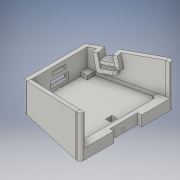
# Autodesk Inventor part: PIUBaseCaseV2
Saved by Autodesk Inventor 2016 (Build 200138000, 138)
## iProperties
Created: 2015-11-04
Part Number: PIUBaseCaseV2
Material: ABS Plastic
Document SubType Name: Modeling
Designer: jonathan
Density: 1.06 g/cm^3
Appearance: Smooth - White
Author: jonathan
Autodesk Inventor part; units mm, degrees
ref_plane "YZ Plane" through (0, 0, 0) normal (1, 0, 0) x (0, 1, 0)
ref_plane "XZ Plane" through (0, 0, 0) normal (0, 1, 0) x (-1, 0, 0)
ref_plane "XY Plane" through (0, 0, 0) normal (0, 0, 1) x (1, 0, 0)
sketch "Sketch1" plane through (0, 0, 0) normal (0, 1, 0) x (-1, 0, 0)
  line L0 (0, 27.305) -> (0, -27.305)
  line L1 (0, 0) -> (-62.23, 0)
  line L2 (-62.23, 41.6814) -> (-62.23, -41.6814)
  line L3 (0, 27.305) -> (-62.23, 41.6814)
  line L4 (0, -27.305) -> (-62.23, -41.6814)
  line L5 (0, -27.305) -> (3.81, -27.305)
  line L6 (3.81, -27.305) -> (3.81, -31.115)
  line L7 (3.81, -31.115) -> (0, -31.115)
  line L8 (0, -31.115) -> (0, -27.305)
  line L9 (0, 27.305) -> (3.81, 27.305)
  line L10 (3.81, 27.305) -> (3.81, 31.115)
  line L11 (3.81, 31.115) -> (0, 31.115)
  line L12 (0, 31.115) -> (0, 27.305)
  line L13 (-62.23, -41.6814) -> (-66.04, -41.6814)
  line L14 (-66.04, -41.6814) -> (-66.04, -45.4914)
  line L15 (-66.04, -45.4914) -> (-62.23, -45.4914)
  line L16 (-62.23, -45.4914) -> (-62.23, -41.6814)
  line L17 (-62.23, 41.6814) -> (-66.04, 41.6814)
  line L18 (-66.04, 41.6814) -> (-66.04, 45.4914)
  line L19 (-66.04, 45.4914) -> (-62.23, 45.4914)
  line L20 (-62.23, 45.4914) -> (-62.23, 41.6814)
  line L21 (3.81, 27.305) -> (3.81, -27.305)
  line L22 (0, -31.115) -> (-62.23, -45.4914)
  line L23 (-66.04, -41.6814) -> (-66.04, 41.6814)
  line L24 (-62.23, 45.4914) -> (0, 31.115)
  dimension "d0" = 54.61
  dimension "d1" = 62.23
  dimension "d2" = 83.3628
  dimension "d3" = 3.81
  dimension "d4" = 3.81
  dimension "d5" = 3.81
  dimension "d6" = 3.81
  dimension "d7" = 3.81
  dimension "d8" = 3.81
  dimension "d9" = 3.81
  dimension "d10" = 3.81
  constraints: 50 end point, 8 parallel, 5 horizontal, 4 perpendicular, 2 midpoint, 2 vertical, 1 coincident
  measures "d0" distance of L0.start L0.end
  measures "d1" distance of L1.end L1.start
  measures "d2" distance of L2.start L2.end
  measures "d3" distance of L6.end L7.end
  measures "d4" distance of L5.end L6.end
  measures "d5" distance of L11.end L10.end
  measures "d6" distance of L10.end L9.end
  measures "d7" distance of L15.end L14.end
  measures "d8" distance of L14.end L13.end
  measures "d9" distance of L18.end L19.end
  measures "d10" distance of L17.end L18.end
extrude "Extrusion1" add sketch "Sketch1" along normal blind 3.81 contours L0 L1 L2 L3 | L0 L4 L2 L1
sketch "Sketch2" plane through (0, 0, 0) normal (0, -1, 0) x (1, 0, 0)
  line L0 (0, -27.305) -> (0, 27.305) projected
  line L1 (0, 27.305) -> (-3.81, 27.305)
  line L2 (-3.81, 27.305) -> (-3.81, 31.115)
  line L3 (-3.81, 31.115) -> (0, 31.115)
  line L4 (0, 31.115) -> (0, 27.305)
  line L5 (0, -27.305) -> (-3.81, -27.305)
  line L6 (-3.81, -27.305) -> (-3.81, -31.115)
  line L7 (-3.81, -31.115) -> (0, -31.115)
  line L8 (0, -31.115) -> (0, -27.305)
  line L9 (62.23, 41.6814) -> (62.23, -41.6814) projected
  line L10 (62.23, -41.6814) -> (66.04, -41.6814)
  line L11 (66.04, -41.6814) -> (66.04, -45.4914)
  line L12 (66.04, -45.4914) -> (62.23, -45.4914)
  line L13 (62.23, -45.4914) -> (62.23, -41.6814)
  line L14 (62.23, 41.6814) -> (66.04, 41.6814)
  line L15 (66.04, 41.6814) -> (66.04, 45.4914)
  line L16 (66.04, 45.4914) -> (62.23, 45.4914)
  line L17 (62.23, 45.4914) -> (62.23, 41.6814)
  line L18 (-3.81, 27.305) -> (-3.81, -27.305)
  point P0 (0, 0)
  dimension "d13" = 3.81
  dimension "d14" = 3.81
  dimension "d15" = 3.81
  dimension "d16" = 3.81
  dimension "d17" = 3.81
  dimension "d18" = 3.81
  dimension "d19" = 3.81
  dimension "d20" = 3.81
  constraints: 34 end point, 8 parallel, 4 horizontal, 4 perpendicular
  measures "d13" distance of L2.end L3.end
  measures "d14" distance of L1.end L2.end
  measures "d15" distance of L7.end L6.end
  measures "d16" distance of L6.end L5.end
  measures "d17" distance of L11.end L12.end
  measures "d18" distance of L10.end L11.end
  measures "d19" distance of L16.end L15.end
  measures "d20" distance of L15.end L14.end
extrude "Extrusion2" add sketch "Sketch2" against normal blind 25.4 contours L5 L18 L1 L0 | L8 L7 L6 L5 | L1 L2 L3 L4
sketch "Sketch3" plane through (0, 0, 0) normal (0, -1, 0) x (1, 0, 0)
  line L0 (62.23, 41.6814) -> (62.23, -41.6814) projected
  line L1 (62.23, -41.6814) -> (66.04, -41.6814)
  line L2 (66.04, -41.6814) -> (66.04, -45.4914)
  line L3 (66.04, -45.4914) -> (62.23, -45.4914)
  line L4 (62.23, -45.4914) -> (62.23, -41.6814)
  line L5 (62.23, 41.6814) -> (66.04, 41.6814)
  line L6 (66.04, 41.6814) -> (66.04, 45.4914)
  line L7 (66.04, 45.4914) -> (62.23, 45.4914)
  line L8 (62.23, 45.4914) -> (62.23, 41.6814)
  line L9 (66.04, -41.6814) -> (66.04, 41.6814)
  point P0 (0, 0)
  dimension "d23" = 3.81
  dimension "d24" = 3.81
  dimension "d25" = 3.81
  dimension "d26" = 3.81
  constraints: 18 end point, 4 parallel, 2 horizontal, 2 perpendicular
  measures "d23" distance of L2.end L3.end
  measures "d24" distance of L1.end L2.end
  measures "d25" distance of L7.end L6.end
  measures "d26" distance of L6.end L5.end
extrude "Extrusion3" add sketch "Sketch3" against normal blind 38.1
sketch "Sketch4" plane through (0, 3.81, 0) normal (0, 1, 0) x (1, 0, 0)
  point P0 (0, 0)
sketch "Sketch5" plane through (0, 0, 27.305) normal (-0.2250919, 0, 0.9743375) x (0.9743375, 0, 0.2250919)
  line L0 (0, 3.81) -> (63.869, 3.81) projected
  line L1 (0, 0) -> (0, 3.81) projected
  line L2 (63.869, 3.81) -> (0, 3.81)
  line L3 (0, 3.81) -> (0, 0)
  line L4 (0, 0) -> (63.869, 0)
  line L5 (63.869, 0) -> (63.869, 3.81)
  line L6 (63.869, 3.81) -> (63.869, 38.1)
  line L7 (0, 3.81) -> (0, 25.4)
  line L8 (0, 25.4) -> (63.869, 38.1)
  point P0 (-6.1461, 0)
  dimension "d29" = 34.29
  dimension "d34" = 21.59
  constraints: 14 end point, 2 parallel, 2 vertical, 1 horizontal, 1 perpendicular
  measures "d29" distance of L0.end L6.end
  measures "d34" distance of L2.end L7.end
extrude "Extrusion4" add sketch "Sketch5" along normal blind 3.81
sketch "Sketch6" plane through (0, 0, 0) normal (0, -1, 0) x (1, 0, 0)
  line L0 (62.23, 41.6814) -> (62.23, -41.6814) projected
  line L1 (62.23, 45.4914) -> (62.23, 41.6814) projected
  line L2 (62.23, 41.6814) -> (62.23, 45.4914)
  line L3 (-0.4344, 31.115) -> (61.3724, 45.3936) projected
  line L4 (62.23, 45.4914) -> (61.3724, 45.3936)
  line L5 (61.3724, 45.3936) -> (62.23, 41.6814)
  point P0 (0, 0)
  constraints: 6 end point, 1 collinear, 1 perpendicular
extrude "Extrusion5" add sketch "Sketch6" against normal blind 38.1
sketch "Sketch7" plane through (0, 0, -27.305) normal (-0.2250919, 0, -0.9743375) x (-0.9743375, 0, 0.2250919)
  point P0 (6.1461, 0)
sketch "Sketch8" plane through (0, 0, -27.305) normal (-0.2250919, 0, -0.9743375) x (-0.9743375, 0, 0.2250919)
  line L0 (-63.869, 0) -> (-63.869, 3.81) projected
  line L1 (-63.869, 3.81) -> (-63.869, 38.1)
  line L2 (-63.869, 3.81) -> (0, 3.81) projected
  line L3 (0, 3.81) -> (0, 25.4)
  line L4 (0, 3.81) -> (-63.869, 3.81)
  line L5 (-63.869, 38.1) -> (0, 25.4)
  point P0 (6.1461, 0)
  dimension "d35" = 34.29
  dimension "d36" = 21.59
  constraints: 8 end point, 2 vertical, 1 collinear
  measures "d35" distance of L0.end L1.end
  measures "d36" distance of L2.end L3.end
extrude "Extrusion6" add sketch "Sketch8" along normal blind 3.81
sketch "Sketch9" plane through (0, 0, 0) normal (0, -1, 0) x (1, 0, 0)
  line L0 (62.23, -45.4914) -> (62.23, -41.6814) projected
  line L1 (-0.4344, -31.115) -> (-3.81, -31.115) projected
  line L2 (-3.81, -31.115) -> (0, -31.115) projected
  line L3 (-0.4344, -31.115) -> (0, -31.115)
  line L4 (0, 27.305) -> (0, -27.305) projected
  line L5 (0, -31.115) -> (0, -27.305)
  line L6 (0, -27.305) -> (62.23, -41.6814)
  line L7 (62.23, -41.6814) -> (61.3724, -45.3936) projected
  line L8 (62.23, -45.4914) -> (61.3724, -45.3936)
  line L9 (61.3724, -45.3936) -> (-0.4344, -31.115)
  line L10 (-0.8576, -31.0172) -> (61.3724, -45.3936) projected
  point P0 (0, 0)
  constraints: 10 end point, 1 collinear, 1 horizontal, 1 perpendicular
extrude "Extrusion7" add sketch "Sketch9" against normal blind 3.81 contours L7 L9 L2 L5 L6
sketch "Sketch10" plane through (0, 0, 0) normal (0, -1, 0) x (1, 0, 0)
  line L0 (0, -27.305) -> (62.23, -41.6814) projected
  line L1 (62.23, -41.6814) -> (62.23, -45.4914)
  line L2 (-0.4344, -31.115) -> (61.3724, -45.3936) projected
  line L3 (62.23, -45.4914) -> (61.3724, -45.3936)
  line L4 (62.23, -41.6814) -> (61.3724, -45.3936) projected
  line L5 (61.3724, -45.3936) -> (62.23, -41.6814)
  point P0 (0, 0)
  constraints: 6 end point, 1 collinear, 1 vertical
extrude "Extrusion8" add sketch "Sketch10" against normal blind 38.1
sketch "Sketch11" plane through (0, 3.81, 0) normal (0, 1, 0) x (1, 0, 0)
  line L0 (62.23, 41.6814) -> (0, 27.305) projected
  line L1 (62.23, -41.6814) -> (62.23, 41.6814) projected
  line L2 (62.23, 41.6814) -> (62.23, -41.6814)
  line L3 (0, -27.305) -> (62.23, -41.6814) projected
  line L4 (62.23, -41.6814) -> (0, -27.305)
  line L5 (0, 27.305) -> (0, -27.305)
  line L6 (62.23, 41.6814) -> (62.23, -41.6814) projected
  line L7 (62.23, 41.6814) -> (0, 27.305)
  line L8 (62.23, 41.6814) -> (58.277, 36.7118)
  line L9 (62.23, 41.6814) -> (68.58, 41.6814) construction
  line L10 (62.23, -41.6814) -> (58.277, -36.7118)
  line L11 (62.23, -41.6814) -> (68.58, -41.6814) construction
  line L12 (0, 27.305) -> (4.9703, 23.3529)
  line L13 (0, 27.305) -> (6.35, 27.305) construction
  line L14 (0, -27.305) -> (4.9703, -23.3529)
  line L15 (0, -27.305) -> (6.35, -27.305) construction
  line L16 (4.9703, -23.3529) -> (4.9703, 23.3529)
  line L17 (58.277, 36.7118) -> (4.9703, 23.3529)
  line L18 (58.277, -36.7118) -> (58.277, 36.7118)
  line L19 (58.277, -36.7118) -> (4.9703, -23.3529)
  line L20 (62.23, -41.6814) -> (113.03, -41.6814)
  point P0 (0, 0)
  dimension "d43" = 6.35
  dimension "d44" = 128.5
  dimension "d45" = 6.35
  dimension "d46" = 128.5
  dimension "d47" = 6.35
  dimension "d48" = 38.49
  dimension "d49" = 6.35
  dimension "d50" = 38.49
  dimension "d53" = 50.8
  constraints: 34 end point, 5 horizontal, 4 equal length, 2 vertical, 1 collinear
  measures "d43" distance of L0.start L8.end
  measures "d44" angle of L8 L9
  measures "d45" distance of L1.start L10.end
  measures "d46" angle of L11 L10
  measures "d47" distance of L0.end L12.end
  measures "d48" angle of L12 L13
  measures "d49" distance of L3.start L14.end
  measures "d50" angle of L15 L14
  measures "d53" distance of L1.start L20.end
extrude "Extrusion9" add sketch "Sketch11" along normal blind 3.81 contours L8 L17 L12 L0 | L1 L10 L18 L8 | L12 L16 L14 L5 | L3 L14 L19 L10
sketch "Sketch12" plane through (66.04, 0, 45.4914) normal (1, 0, 0) x (0, 0, -1)
  line L0 (45.4914, 0) -> (45.4914, 3.81)
  line L1 (8.7796, 3.81) -> (82.2032, 3.81) projected
  line L2 (87.1728, 7.62) -> (3.81, 7.62) projected
  line L3 (45.4914, 7.62) -> (45.4914, 3.81)
  line L4 (56.2864, 11.43) -> (56.2864, 7.62)
  line L5 (56.2864, 7.62) -> (34.6964, 7.62)
  line L6 (3.81, 7.62) -> (0, 7.62)
  line L7 (0, 0) -> (0, 38.1) projected
  line L8 (8.7796, 7.62) -> (22.1385, 7.62) projected
  line L9 (8.7796, 7.62) -> (17.6696, 7.62)
  line L10 (18.1864, 7.62) -> (72.7964, 7.62) projected
  line L11 (8.7796, 7.62) -> (33.6716, 7.62)
  line L12 (33.6716, 7.62) -> (34.6964, 7.62)
  line L13 (56.2864, 11.43) -> (34.6964, 11.43)
  line L14 (82.2032, 7.62) -> (8.7796, 7.62) projected
  line L15 (8.7796, 7.62) -> (17.6696, 7.62)
  line L16 (17.6696, 7.62) -> (17.6696, 13.97)
  line L17 (34.6964, 11.43) -> (34.6964, 7.62)
  line L18 (34.6964, 7.62) -> (29.6164, 7.62)
  line L19 (29.6164, 7.62) -> (29.6164, 13.97)
  line L20 (29.6164, 13.97) -> (17.6696, 13.97)
  dimension "d54" = 21.59
  dimension "d55" = 3.81
  dimension "d58" = 8.89
  dimension "d59" = 24.892
  dimension "d62" = 8.89
  dimension "d63" = 6.35
  dimension "d64" = 5.08
  dimension "d65" = 6.35
  dimension "d66" = 21.59
  constraints: 30 end point, 5 point on line, 3 midpoint, 2 horizontal, 2 perpendicular, 1 collinear, 1 parallel, 1 vertical
  measures "d54" distance of L4.end L5.end
  measures "d55" distance of L4.start L4.end
  measures "d58" distance of L8.start L9.end
  measures "d59" distance of L8.start L11.end
  measures "d62" distance of L8.start L15.end
  measures "d63" distance of L15.end L16.end
  measures "d64" distance of L5.end L18.end
  measures "d65" distance of L18.end L19.end
  measures "d66" distance of L4.start L13.end
extrude "Extrusion10" cut sketch "Sketch12" against normal blind 6.35
sketch "Sketch13" plane through (-3.81, 0, -31.115) normal (-1, 0, 0) x (0, 0, 1)
  line L0 (22.225, 11.43) -> (40.005, 11.43)
  line L1 (40.005, 11.43) -> (40.005, 7.62)
  line L2 (22.225, 7.62) -> (22.225, 11.43)
  line L3 (7.7621, 3.81) -> (54.4679, 3.81) projected
  line L4 (40.005, 7.62) -> (22.225, 7.62)
  line L5 (58.42, 7.62) -> (3.81, 7.62) projected
  point P0 (31.115, 0)
  point P1 (31.115, 3.81)
  point P2 (31.115, 7.62)
  dimension "d67" = 17.78
  dimension "d68" = 3.81
  constraints: 8 end point, 3 midpoint, 2 horizontal, 1 parallel, 1 perpendicular
  measures "d67" distance of L1.end L2.start
  measures "d68" distance of L0.end L1.end
extrude "Extrusion11" cut sketch "Sketch13" against normal blind 25.4
sketch "Sketch14" plane through (-3.81, 0, -31.115) normal (-1, 0, 0) x (0, 0, 1)
  line L0 (31.115, 25.4) -> (31.115, 21.59)
  line L1 (0, 25.4) -> (62.23, 25.4) projected
  line L2 (31.115, 21.59) -> (24.765, 21.59)
  line L3 (24.765, 21.59) -> (24.765, 17.78)
  line L4 (24.765, 17.78) -> (37.465, 17.78)
  line L5 (37.465, 17.78) -> (37.465, 21.59)
  line L6 (37.465, 21.59) -> (31.115, 21.59)
  point P0 (31.115, 0)
  dimension "d73" = 3.81
  dimension "d74" = 6.35
  dimension "d75" = 3.81
  dimension "d76" = 12.7
  dimension "d77" = 3.81
  constraints: 12 end point, 2 perpendicular, 1 horizontal, 1 midpoint, 1 point on line, 1 vertical
  measures "d73" distance of L0.start L0.end
  measures "d74" distance of L0.end L2.end
  measures "d75" distance of L2.end L3.end
  measures "d76" distance of L3.end L4.end
  measures "d77" distance of L4.end L5.end
extrude "Extrusion12" cut sketch "Sketch14" against normal blind 25.4
sketch "Sketch16" plane through (0, 38.1, 0) normal (0, 1, 0) x (1, 0, 0)
  line L0 (62.23, 41.6814) -> (62.23, -41.6814) projected
  line L1 (66.04, -45.4914) -> (66.04, 45.4914) projected
  line L2 (62.23, 41.6814) -> (66.04, 41.6814)
  line L3 (66.04, 41.6814) -> (66.04, -41.6814)
  line L4 (66.04, -41.6814) -> (62.23, -41.6814)
  line L5 (62.23, -41.6814) -> (62.23, 41.6814)
  point P0 (0, 0)
  dimension "d80" = 83.3628
  constraints: 8 end point, 2 parallel, 1 horizontal, 1 perpendicular, 1 point on line
  measures "d80" distance between parallel lines of L2 L4
extrude "Extrusion13" cut sketch "Sketch16" against normal blind 30.48
sketch "Sketch17" plane through (0, 7.62, 0) normal (0, 1, 0) x (1, 0, 0)
  line L0 (62.23, -6.35) -> (66.04, -6.35)
  line L1 (66.04, -6.35) -> (66.04, 6.35)
  line L2 (66.04, 6.35) -> (62.23, 6.35)
  line L3 (62.23, 6.35) -> (62.23, -6.35)
  line L4 (66.04, 41.6814) -> (66.04, -41.6814) projected
  line L5 (62.23, 0) -> (62.23, -12.319)
  line L6 (62.23, -12.319) -> (66.04, -12.319)
  line L7 (66.04, -12.319) -> (66.04, 6.35)
  line L8 (66.04, 45.4914) -> (66.04, -45.4914) projected
  line L9 (62.23, 6.35) -> (62.23, 12.065)
  line L10 (62.23, 12.065) -> (66.04, 12.065)
  line L11 (66.04, 12.065) -> (66.04, 6.35)
  point P0 (0, 0)
  point P1 (66.04, 0)
  dimension "d83" = 3.81
  dimension "d84" = 12.7
  dimension "d143" = 12.319
  dimension "d144" = 3.81
  dimension "d145" = 5.715
  dimension "d146" = 3.81
  constraints: 20 end point, 3 midpoint, 2 parallel, 2 point on line, 2 vertical, 1 collinear, 1 horizontal, 1 perpendicular
  measures "d83" distance of L2.end L1.end
  measures "d84" distance of L1.end L0.end
  measures "d143" distance of L5.start L5.end
  measures "d144" distance of L5.end L6.end
  measures "d145" distance of L2.end L9.end
  measures "d146" distance of L9.end L10.end
extrude "Extrusion14" cut sketch "Sketch17" against normal blind 7.62 contours L3 L2 L1 L0
sketch "Sketch19" plane through (0, 0, 0) normal (0, -1, 0) x (1, 0, 0)
  line L0 (66.04, 45.4914) -> (62.23, 45.4914) projected
  line L1 (62.23, 45.4914) -> (61.3724, 45.3936) projected
  line L2 (66.04, 45.4914) -> (62.23, 45.4914)
  line L3 (62.23, 45.4914) -> (61.3724, 45.3936)
  line L4 (-3.81, 31.115) -> (-0.4344, 31.115) projected
  line L5 (61.3724, 45.3936) -> (-0.4344, 31.115)
  line L6 (-3.81, 31.115) -> (-3.81, -31.115) projected
  line L7 (-0.4344, 31.115) -> (-3.81, 31.115)
  line L8 (-3.81, 31.115) -> (-3.81, -31.115)
  line L9 (-3.81, -31.115) -> (-0.4344, -31.115) projected
  line L10 (-3.81, -31.115) -> (-0.4344, -31.115)
  line L11 (-0.8576, -31.0172) -> (61.3724, -45.3936) projected
  line L12 (-0.4344, -31.115) -> (61.3724, -45.3936)
  line L13 (62.23, -45.4914) -> (66.04, -45.4914) projected
  line L14 (61.3724, -45.3936) -> (62.23, -45.4914)
  line L15 (66.04, -45.4914) -> (66.04, -6.35) projected
  line L16 (62.23, -45.4914) -> (66.04, -45.4914)
  line L17 (66.04, -45.4914) -> (66.04, -6.35)
  line L18 (66.04, -6.35) -> (62.23, -6.35)
  line L19 (62.23, -6.35) -> (62.23, 6.35) projected
  line L20 (62.23, -6.35) -> (62.23, 6.35)
  line L21 (62.23, 6.35) -> (66.04, 6.35)
  line L22 (66.04, 6.35) -> (66.04, 45.4914)
  point P0 (0, 0)
  constraints: 28 end point, 5 perpendicular, 4 collinear, 2 parallel, 1 horizontal
extrude "Extrusion15" add sketch "Sketch19" along normal blind 2.54
sketch "Sketch20" plane through (62.23, 7.62, 6.35) normal (1, 0, 0) x (0, 0, -1)
  line L0 (6.35, -6.985) -> (6.35, -10.16)
  line L1 (12.7, -10.16) -> (0, -10.16) projected
  circle A0 centre (6.35, -6.985) radius 1.4097
  point P0 (6.35, -7.62)
  dimension "d128" = 3.175
  dimension "d129" = 2.8194
  constraints: 2 end point, 1 centre point, 1 coincident, 1 midpoint, 1 vertical
  measures "d128" distance of L0.end L0.start
  measures "d129" diameter of A0
extrude "Extrusion16" cut sketch "Sketch20" against normal blind 8.89
sketch "Sketch21" plane through (0, 3.81, 0) normal (0, 1, 0) x (1, 0, 0)
  line L0 (62.23, 6.35) -> (62.23, -6.35) projected
  line L1 (62.23, 0) -> (53.34, 0)
  line L2 (48.26, -3.175) -> (53.34, -3.175)
  line L3 (53.34, -3.175) -> (53.34, 3.175)
  line L4 (53.34, 3.175) -> (48.26, 3.175)
  line L5 (48.26, 3.175) -> (48.26, -3.175)
  point P0 (0, 0)
  dimension "d132" = 8.89
  dimension "d133" = 5.08
  dimension "d134" = 6.35
  constraints: 10 end point, 2 horizontal, 2 midpoint, 2 parallel, 1 perpendicular
  measures "d132" distance of L1.end L1.start
  measures "d133" distance of L4.end L3.end
  measures "d134" distance of L3.end L2.end
extrude "Extrusion17" cut sketch "Sketch21" against normal blind 8.89
sketch "Sketch24" plane through (0, 7.62, 0) normal (0, 1, 0) x (1, 0, 0)
  line L0 (62.23, -6.35) -> (66.04, -6.35)
  line L1 (66.04, -6.35) -> (66.04, 6.35)
  line L2 (66.04, 6.35) -> (62.23, 6.35)
  line L3 (62.23, 6.35) -> (62.23, -6.35)
  line L4 (66.04, 42.3164) -> (66.04, -42.3164)
  line L5 (62.23, 0) -> (62.23, -12.954)
  line L6 (62.23, -12.954) -> (66.04, -12.954)
  line L7 (66.04, -12.954) -> (66.04, 6.35)
  line L8 (66.04, 47.5234) -> (66.04, -43.4594)
  line L9 (62.23, 6.35) -> (62.23, 14.097)
  line L10 (62.23, 14.097) -> (66.04, 14.097)
  line L11 (66.04, 14.097) -> (66.04, 6.35)
  line L12 (62.23, 0) -> (66.04, 0)
  line L13 (62.23, 1.4097) -> (62.23, -1.4097) projected
  point P0 (0, 0)
  point P1 (66.04, 21.082)
  dimension "d147" = 3.81
  dimension "d148" = 12.7
  dimension "d149" = 12.954
  dimension "d150" = 3.81
  dimension "d151" = 7.747
  dimension "d152" = 3.81
  constraints: 26 end point, 3 midpoint, 3 point on line, 2 parallel, 2 perpendicular, 2 vertical, 1 collinear, 1 horizontal
  measures "d147" distance of L2.end L11.end
  measures "d148" distance of L11.end L0.end
  measures "d149" distance of L5.start L5.end
  measures "d150" distance of L5.end L6.end
  measures "d151" distance of L2.end L10.start
  measures "d152" distance of L10.start L10.end
extrude "Extrusion19" cut sketch "Sketch24" against normal blind 25.4 contours L0 L4 L6 L5 | L2 L9 L10 L4
sketch "Sketch25" plane through (0, 0, -27.305) normal (0.2250919, 0, 0.9743375) x (0.9743375, 0, -0.2250919)
  line L0 (0, 25.4) -> (11.2105, 27.6291)
  line L1 (11.2105, 27.6291) -> (13.6874, 15.173)
  line L2 (11.2105, 27.6291) -> (7.4737, 26.8861)
  line L3 (13.6874, 15.173) -> (26.1435, 17.6498)
  line L4 (11.2105, 27.6291) -> (23.6667, 30.106)
  line L5 (0, 25.4) -> (63.869, 38.1) projected
  line L6 (23.6667, 30.106) -> (26.1435, 17.6498)
  line L7 (7.4737, 26.8861) -> (10.6936, 10.6931)
  line L8 (10.6936, 10.6931) -> (30.6234, 14.6561)
  line L9 (30.6234, 14.6561) -> (27.4035, 30.849)
  line L10 (23.6667, 30.106) -> (27.4035, 30.849)
  point P0 (-6.1461, 0)
  dimension "d157" = 11.43
  dimension "d158" = 12.7
  dimension "d161" = 3.81
  dimension "d168" = 12.7
  dimension "d169" = 12.7
  dimension "d170" = 16.51
  dimension "d171" = 20.32
  dimension "d172" = 16.51
  constraints: 20 end point, 3 parallel, 2 collinear, 1 perpendicular, 1 point on line
  measures "d157" distance of L0.start L0.end
  measures "d158" distance of L0.end L1.end
  measures "d161" distance of L0.end L2.end
  measures "d168" distance of L1.end L3.end
  measures "d169" distance of L0.end L4.end
  measures "d170" distance of L2.end L7.end
  measures "d171" distance of L7.end L8.end
  measures "d172" distance of L8.end L9.end
extrude "Extrusion20" add sketch "Sketch25" along normal blind 3.81
sketch "Sketch26" plane through (0.8576, 0, -23.5928) normal (0.2250919, 0, 0.9743375) x (0.9743375, 0, -0.2250919)
  line L0 (26.1435, 17.6498) -> (26.8865, 13.913)
  line L1 (26.1435, 17.6498) -> (29.9535, 17.6498) construction
  line L2 (30.6234, 14.6561) -> (27.4035, 30.849) projected
  line L3 (26.1435, 17.6498) -> (29.8803, 18.3929)
  line L4 (10.6936, 10.6931) -> (30.6234, 14.6561) projected
  line L5 (29.8803, 18.3929) -> (30.6234, 14.6561)
  line L6 (26.1435, 17.6498) -> (13.6874, 15.173) projected
  line L7 (26.1435, 17.6498) -> (29.8803, 18.3929)
  line L8 (30.6234, 14.6561) -> (26.8865, 13.913)
  line L9 (26.1435, 17.6498) -> (26.8865, 13.913)
  line L10 (30.6234, 14.6561) -> (29.8803, 18.3929)
  point P0 (-6.1461, 0)
  dimension "d173" = 3.81
  dimension "d175" = 3.81
  constraints: 16 end point, 3 collinear, 2 parallel, 1 horizontal
  measures "d173" distance of L0.start L0.end
  measures "d175" distance of L0.start L3.end
extrude "Extrusion21" cut sketch "Sketch26" against normal blind 3.81
sketch "Sketch28" plane through (0.8576, 0, -23.5928) normal (0.2250919, 0, 0.9743375) x (0.9743375, 0, -0.2250919)
  line L0 (27.4035, 30.849) -> (7.4737, 26.8861) projected
  line L1 (7.4737, 26.8861) -> (10.6936, 10.6931)
  line L2 (10.6936, 10.6931) -> (26.8865, 13.913)
  line L3 (26.8865, 13.913) -> (26.1435, 17.6498) projected
  line L4 (26.8865, 13.913) -> (26.1435, 17.6498)
  line L5 (26.1435, 17.6498) -> (29.8803, 18.3929) projected
  line L6 (26.1435, 17.6498) -> (29.8803, 18.3929)
  line L7 (29.8803, 18.3929) -> (27.4035, 30.849)
  line L8 (27.4035, 30.849) -> (7.4737, 26.8861)
  line L9 (7.4737, 26.8861) -> (10.6936, 10.6931) projected
  line L10 (7.4737, 26.8861) -> (11.1607, 27.6192)
  line L11 (11.1607, 27.6192) -> (11.8988, 23.9073)
  line L12 (27.4035, 30.849) -> (23.6916, 30.1109)
  line L13 (23.6916, 30.1109) -> (24.4297, 26.399)
  line L14 (29.8803, 18.3929) -> (27.4035, 30.849) projected
  line L15 (11.8988, 23.9073) -> (24.4297, 26.399)
  line L16 (10.6936, 10.6931) -> (14.3806, 11.4263)
  line L17 (14.3806, 11.4263) -> (13.6425, 15.1382)
  line L18 (24.4297, 26.399) -> (26.956, 13.6937)
  line L19 (26.1435, 17.6498) -> (26.1684, 17.6548)
  line L20 (26.8865, 13.913) -> (26.9115, 13.918)
  line L21 (26.9115, 13.918) -> (26.1684, 17.6548)
  line L22 (26.1684, 17.6548) -> (26.1435, 17.6498)
  line L23 (26.1684, 17.6548) -> (13.6425, 15.1382)
  line L24 (11.8988, 23.9073) -> (13.6425, 15.1382)
  line L25 (11.8988, 23.9073) -> (13.6425, 15.1382)
  line L26 (13.6425, 15.1382) -> (26.1684, 17.6548)
  line L27 (26.1684, 17.6548) -> (24.4297, 26.399)
  line L28 (24.4297, 26.399) -> (11.8988, 23.9073)
  line L29 (13.6425, 15.1382) -> (14.3806, 11.4263)
  line L30 (10.6936, 10.6931) -> (26.8865, 13.913) projected
  line L31 (14.3806, 11.4263) -> (26.8865, 13.913)
  point P0 (-6.1461, 0)
  dimension "d178" = 3.7592
  dimension "d179" = 3.7846
  dimension "d180" = 3.7846
  dimension "d181" = 3.7846
  dimension "d182" = 3.7592
  dimension "d183" = 3.7846
  dimension "d184" = 12.954
  dimension "d185" = 0.0254
  constraints: 52 end point, 6 collinear, 5 perpendicular, 4 parallel, 2 point on line
  measures "d178" distance of L0.end L10.end
  measures "d179" distance of L10.end L11.end
  measures "d180" distance of L0.start L12.end
  measures "d181" distance of L12.end L13.end
  measures "d182" distance of L1.end L16.end
  measures "d183" distance of L16.end L17.end
  measures "d184" distance of L13.end L18.end
  measures "d185" distance of L2.end L20.end
extrude "Extrusion23" add sketch "Sketch28" along normal blind 1 contours L7 L5 L18 L13 L0 | L11 L24 L17 L2 L1 L0 | L3 L2 L17 L23
sketch "Sketch29" plane through (0.8576, 0, -23.5928) normal (0.2250919, 0, 0.9743375) x (0.9743375, 0, -0.2250919)
  line L0 (11.1607, 27.6192) -> (11.634, 27.7134)
  line L1 (23.6916, 30.1109) -> (11.1607, 27.6192) projected
  line L2 (23.209, 30.015) -> (23.6916, 30.1109)
  line L3 (11.634, 27.7134) -> (12.922, 21.2362)
  line L4 (11.1607, 27.6192) -> (13.6425, 15.1382) projected
  line L5 (23.209, 30.015) -> (24.4969, 23.5378)
  line L6 (12.922, 21.2362) -> (24.4969, 23.5378)
  line L7 (11.634, 27.7134) -> (23.209, 30.015)
  point P0 (-6.1461, 0)
  dimension "d190" = 0.4826
  dimension "d191" = 0.4826
  dimension "d192" = 6.604
  dimension "d193" = 6.604
  constraints: 12 end point, 2 collinear, 2 parallel
  measures "d190" distance of L0.start L0.end
  measures "d191" horizontal distance of L1.start L2.start
  measures "d192" distance of L0.end L3.end
  measures "d193" distance of L2.start L5.end
extrude "Extrusion24" cut sketch "Sketch29" against normal blind 25.4
sketch "Sketch30" plane through (0.8576, 0, -23.5928) normal (0.2250919, 0, 0.9743375) x (0.9743375, 0, -0.2250919)
  line L0 (13.6425, 15.1382) -> (13.3889, 16.4132)
  line L1 (11.1607, 27.6192) -> (13.6425, 15.1382) projected
  line L2 (26.1684, 17.6548) -> (25.9149, 18.9298)
  line L3 (26.1684, 17.6548) -> (23.6916, 30.1109) projected
  line L4 (25.9149, 18.9298) -> (13.3889, 16.4132)
  line L5 (25.9149, 18.9298) -> (25.5966, 20.5305)
  line L6 (13.3889, 16.4132) -> (13.0707, 18.0139)
  line L7 (13.0707, 18.0139) -> (25.5966, 20.5305)
  point P0 (-6.1461, 0)
  dimension "d196" = 1.3
  dimension "d197" = 1.3
  dimension "d198" = 1.632
  dimension "d199" = 1.632
  constraints: 12 end point, 4 collinear
  measures "d196" distance of L0.start L0.end
  measures "d197" distance of L2.start L2.end
  measures "d198" distance of L2.end L5.end
  measures "d199" distance of L0.end L6.end
extrude "Extrusion25" cut sketch "Sketch30" against normal blind 2.54
sketch "Sketch32" plane through (0, 7.62, 0) normal (0, 1, 0) x (1, 0, 0)
  line L0 (62.23, -41.6814) -> (0, -27.305) projected
  line L1 (62.23, -41.6814) -> (62.23, -35.3314)
  line L2 (62.23, -35.3314) -> (55.88, -35.3314)
  line L3 (55.88, -35.3314) -> (55.88, -40.2144)
  line L4 (62.23, -41.6814) -> (55.88, -40.2144)
  line L5 (0, 0) -> (58.277, 0)
  line L6 (58.277, -36.7118) -> (58.277, 36.7118) projected
  line L7 (62.23, 41.6814) -> (0, 27.305)
  line L8 (62.23, 41.6814) -> (62.23, 35.3314)
  line L9 (62.23, 35.3314) -> (55.88, 35.3314)
  line L10 (55.88, 35.3314) -> (55.88, 40.2144)
  line L11 (62.23, 41.6814) -> (55.88, 40.2144)
  line L12 (0, 27.305) -> (0, 20.955)
  line L13 (0, 8.89) -> (0, 27.305) projected
  line L14 (0, 20.955) -> (6.35, 20.955)
  line L15 (6.35, 20.955) -> (6.35, 28.772)
  line L16 (6.35, 20.955) -> (14.167, 20.955) construction
  line L17 (6.35, 28.772) -> (0, 27.305)
  line L18 (0, -27.305) -> (0, -20.955)
  line L19 (0, -20.955) -> (6.35, -20.955)
  line L20 (6.35, -20.955) -> (6.35, -28.772)
  line L21 (6.35, -20.955) -> (14.167, -20.955) construction
  line L22 (6.35, -28.772) -> (0, -27.305)
  dimension "d204" = 6.35
  dimension "d205" = 6.35
  dimension "d206" = 6.35
  dimension "d207" = 6.35
  dimension "d208" = 90
  constraints: 40 end point, 9 symmetric about line, 4 perpendicular, 4 point on line, 1 collinear, 1 horizontal, 1 midpoint, 1 vertical
  measures "d204" distance of L0.start L1.end
  measures "d205" distance of L1.end L2.end
  measures "d206" distance of L7.end L12.end
  measures "d207" distance of L12.end L14.end
  measures "d208" angle of L16 L15
extrude "Extrusion26" add sketch "Sketch32" against normal blind 6.35
sketch "Sketch33" plane through (0, 7.62, 0) normal (0, 1, 0) x (1, 0, 0)
  line L0 (4.9703, -20.955) -> (4.9703, 20.955) projected
  line L1 (4.9703, -20.955) -> (0, -20.955)
  line L2 (4.9703, 20.955) -> (0, 20.955)
  line L3 (0, 20.955) -> (0, -20.955)
  line L4 (4.9703, -20.955) -> (4.9703, 20.955)
  line L5 (6.35, -23.6987) -> (55.88, -36.1111) projected
  line L6 (6.35, -23.6987) -> (6.35, -28.7283)
  line L7 (55.88, -36.1111) -> (55.88, -40.2144)
  line L8 (62.23, -41.6814) -> (0, -27.305) projected
  line L9 (6.35, -23.6987) -> (55.88, -36.1111)
  line L10 (6.35, -28.7283) -> (55.88, -40.2144)
  line L11 (4.9703, 0) -> (58.277, 0)
  line L12 (58.277, -35.3314) -> (58.277, 35.3314) projected
  line L13 (4.9703, 20.955) -> (0, 20.955)
  line L14 (6.35, 23.6987) -> (55.88, 36.1111)
  line L15 (6.35, 23.6987) -> (6.35, 28.7283)
  line L16 (55.88, 36.1111) -> (55.88, 40.2144)
  line L17 (62.23, 41.6814) -> (0, 27.305)
  line L18 (6.35, 23.6987) -> (55.88, 36.1111)
  line L19 (6.35, 28.7283) -> (55.88, 40.2144)
  point P0 (0, 0)
  constraints: 32 end point, 6 symmetric about line, 2 horizontal, 2 midpoint, 2 point on line, 2 vertical, 1 parallel, 1 perpendicular
extrude "Extrusion27" cut sketch "Sketch33" against normal blind 3.81
fillet "Fillet1" radius 3.175 2 edges at (28.3879, 18.0238, -28.9265) (26.9173, 15.7814, -28.5868)
fillet "Fillet2" radius 3.175 4 edges at (-3.81, 11.43, 31.115) (-3.81, 11.43, -31.115) (66.04, 17.78, -45.4914) (66.04, 17.78, 45.4914)
move faces "Move1" translate (0, 2.54, 0) faces at (-2.54, 11.43, -2.9633)
body "Solid1"
